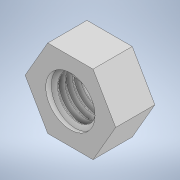
# Autodesk Inventor part: exNut0_3-V01
Saved by Autodesk Inventor 2021.1 (Build 251245010, 245A)
## iProperties
Created: 2020-10-15
Part Number: exNut0_3-V01
Material: Generic
Document SubType Name: Modeling
Designer: robst
Density: 1 g/cm^3
Appearance: Default
Author: robst
Autodesk Inventor part; units mm, degrees
ref_plane "YZ Plane" through (0, 0, 0) normal (1, 0, 0) x (0, 1, 0)
ref_plane "XZ Plane" through (0, 0, 0) normal (0, 1, 0) x (-1, 0, 0)
ref_plane "XY Plane" through (0, 0, 0) normal (0, 0, 1) x (1, 0, 0)
sketch "Sketch1" plane through (0, 0, 0) normal (0, 0, 1) x (1, 0, 0)
  line L0 (-3.6662, 6.35) -> (3.6662, 6.35)
  line L1 (3.6662, 6.35) -> (7.3323, 0)
  line L2 (7.3323, 0) -> (3.6662, -6.35)
  line L3 (3.6662, -6.35) -> (-3.6662, -6.35)
  line L4 (-3.6662, -6.35) -> (-7.3323, 0)
  line L5 (-7.3323, 0) -> (-3.6662, 6.35)
  point P0 (0, 0)
  point P1 (0, 0)
  dimension "d0" = 12.7
  constraints: 12 end point, 1 coincident, 1 horizontal, 13 other
  measures "d0" distance between parallel lines of L3 L0
extrude "Extrusion1" add sketch "Sketch1" along normal blind 6.35
sketch "Sketch2" plane through (0, 0, 6.35) normal (0, 0, 1) x (1, 0, 0)
  circle A0 centre (0, 0) radius 3.9903
  dimension "d3" = 7.9807
  constraints: 1 centre point, 1 coincident
  measures "d3" diameter of A0
extrude "Extrusion2" cut sketch "Sketch2" against normal through all
sketch "Sketch3" plane through (0, 0, 0) normal (1, 0, 0) x (0, 1, 0)
  line L0 (3.9903, 6.35) -> (3.9903, 0) projected
  line L1 (-3.9903, 6.35) -> (3.9903, 6.35) projected
  line L2 (3.9903, 6.35) -> (3.9903, 5.4936)
  line L3 (3.9903, 5.4936) -> (3.3477, 5.8646)
  line L4 (3.3477, 5.979) -> (3.9903, 6.35)
  arc A0 (3.3477, 5.979) -> (3.3477, 5.8646) centre (3.3807, 5.9218) ccw
  line L5 (0, 0) -> (0, 6.35) projected
  dimension "d6" = 60
  dimension "d7" = 0.066
  dimension "d8" = 3.3147
  dimension "d17" = 0.8564
  constraints: 6 end point, 2 point on circle, 2 tangent, 1 centre point, 1 equal length, 1 point on line
  measures "d6" angle of L3 L4
  measures "d7" radius of A0
  measures "d8" distance edge to line of A0 L5
  measures "d17" distance of L2.end L0.start
coil "Coil1" sketch "Sketch3" operation add axis through (0, 0, -10) along (0, 0, -1) pitch 1.2095 turns 4.541938 hand right
equation "\"d3\" = b1Major"
equation "\"d7\" = b1RootRadius"
equation "\"d8\" = b1MinorRadius"
equation "\"d9\" = pitch"
equation "\"b1Major\" = 7.98068"
equation "\"b1Minor\" = 6.6294"
equation "\"b1RootRadius\" = 0.06604"
equation "\"b1MinorRadius\" = 0.5 * b1Minor"
equation "\"pitch\" = 1.209524"
body "Solid1"
